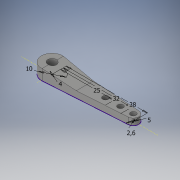
# Autodesk Inventor part: ServoArm 38mm
Saved by Autodesk Inventor 2018.2 (Build 222227000, 227)
## iProperties
Created: 2018-02-17
Part Number: ServoArm 38mm
Material: Generisch
Document SubType Name: Modeling
Designer: JochenAlt
Density: 1 g/cm^3
Appearance: Vorgabe
Author: JochenAlt
Autodesk Inventor part; units mm, degrees
ref_plane "YZ Plane" through (0, 0, 0) normal (1, 0, 0) x (0, 1, 0)
ref_plane "XZ Plane" through (0, 0, 0) normal (0, 1, 0) x (-1, 0, 0)
ref_plane "XY Plane" through (0, 0, 0) normal (0, 0, 1) x (1, 0, 0)
sketch "Skizze1" plane through (0, 0, 0) normal (0, 0, 1) x (1, 0, 0)
  line L0 (0, 7) -> (0, -7) construction
  line L1 (-14.1, 0) -> (49.6, 0) construction
  circle A0 centre (0, 0) radius 2
  circle A1 centre (25, 0) radius 1.3257
  circle A2 centre (32, 0) radius 1.3
  circle A3 centre (38, 0) radius 1.3
  arc A4 (38.1645, -2.4946) -> (38.1645, 2.4946) centre (38, 0) ccw
  arc A5 (0.3289, 4.9892) -> (0.3289, -4.9892) centre (0, 0) ccw
  line L2 (0.3289, 4.9892) -> (38.1645, 2.4946)
  line L3 (0.3289, -4.9892) -> (38.1645, -2.4946)
  line L4 (0.3289, -4.9892) -> (0.3289, -1.9728)
  line L5 (0.3289, 1.9728) -> (0.3289, 4.9892)
  line L6 (0.3289, 1.9728) -> (0.3289, -1.9728)
  dimension "d0" = 25
  dimension "d1" = 32
  dimension "d2" = 38
  dimension "d3" = 5
  dimension "d4" = 2.6
  dimension "d5" = 4
  dimension "d6" = 10
  constraints: 10 end point, 8 point on circle, 6 centre point, 4 tangent, 3 coincident, 3 point on line, 1 collinear, 1 equal radius, 1 vertical
  measures "d0" distance of A1.centre point (0, 0)
  measures "d1" distance of point (0, 0) A2.centre
  measures "d2" distance of A3.centre point (0, 0)
  measures "d3" diameter of A4
  measures "d4" diameter of A3
  measures "d5" diameter of A0
  measures "d6" diameter of A5
extrude "Extrusion1" add sketch "Skizze1" along normal blind 3
extrude "Extrusion2" add sketch "Skizze1" along normal blind 5 contours L6 A0 | A0 L4 A5 L5 picked at (-0.6966, -0.3173)
chamfer "Fase1" distance 15 distance2 2 1 edges at (0.3289, 0, 3) measured on face at (0.8289, 0, 3)
extrude "Extrusion3" cut sketch "Skizze1" along normal blind 5 contours A0 L6 | L6 A0
